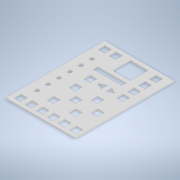
# Autodesk Inventor part: Front Plywood
Saved by Autodesk Inventor 2021.1 (Build 251245000, 245)
## iProperties
Created: 2020-08-02
Part Number: Front Plywood
Material: Generic
Document SubType Name: Modeling
Designer: adick
Density: 1 g/cm^3
Appearance: Default
Author: adick
Autodesk Inventor part; units mm, degrees
ref_plane "YZ Plane" through (0, 0, 0) normal (1, 0, 0) x (0, 1, 0)
ref_plane "XZ Plane" through (0, 0, 0) normal (0, 1, 0) x (-1, 0, 0)
ref_plane "XY Plane" through (0, 0, 0) normal (0, 0, 1) x (1, 0, 0)
sketch "Sketch1" plane through (0, 0, 0) normal (0, 1, 0) x (-1, 0, 0)
  line L0 (0, 0) -> (190, 0)
  line L1 (190, 0) -> (190, -270)
  line L2 (190, -270) -> (0, -270)
  line L3 (0, -270) -> (0, 0)
  line L4 (180, -10) -> (160, -10)
  line L5 (160, -10) -> (160, -30)
  line L6 (160, -30) -> (180, -30)
  line L7 (180, -30) -> (180, -10)
  line L8 (150, -10) -> (130, -10)
  line L9 (130, -10) -> (130, -30)
  line L10 (130, -30) -> (150, -30)
  line L11 (150, -30) -> (150, -10)
  line L12 (120, -10) -> (100, -10)
  line L13 (100, -10) -> (100, -30)
  line L14 (100, -30) -> (120, -30)
  line L15 (120, -30) -> (120, -10)
  line L16 (90, -10) -> (70, -10)
  line L17 (70, -10) -> (70, -30)
  line L18 (70, -30) -> (90, -30)
  line L19 (90, -30) -> (90, -10)
  line L20 (60, -10) -> (40, -10)
  line L21 (40, -10) -> (40, -30)
  line L22 (40, -30) -> (60, -30)
  line L23 (60, -30) -> (60, -10)
  line L24 (28.2524, -10) -> (8.2524, -10)
  line L25 (8.2524, -10) -> (8.2524, -30)
  line L26 (8.2524, -30) -> (28.2524, -30)
  line L27 (28.2524, -30) -> (28.2524, -10)
  circle A0 centre (165, -60) radius 6
  circle A1 centre (165, -90) radius 6
  circle A2 centre (165, -120) radius 6
  circle A3 centre (165, -150) radius 6
  circle A4 centre (165, -180) radius 6
  circle A5 centre (165, -210) radius 6
  line L28 (180, -260) -> (160, -260)
  line L29 (160, -260) -> (160, -240)
  line L30 (160, -240) -> (180, -240)
  line L31 (180, -240) -> (180, -260)
  line L32 (150, -260) -> (130, -260)
  line L33 (130, -260) -> (130, -240)
  line L34 (130, -240) -> (150, -240)
  line L35 (150, -240) -> (150, -260)
  line L36 (130, -50) -> (110, -50)
  line L37 (110, -50) -> (110, -70)
  line L38 (110, -70) -> (130, -70)
  line L39 (130, -70) -> (130, -50)
  line L40 (100, -80) -> (80, -80)
  line L41 (80, -80) -> (80, -100)
  line L42 (80, -100) -> (100, -100)
  line L43 (100, -100) -> (100, -80)
  line L44 (70, -70) -> (50, -70)
  line L45 (50, -70) -> (50, -50)
  line L46 (50, -50) -> (70, -50)
  line L47 (70, -50) -> (70, -70)
  line L48 (70, -110) -> (50, -110)
  line L49 (50, -110) -> (50, -130)
  line L50 (50, -130) -> (70, -130)
  line L51 (70, -130) -> (70, -110)
  line L52 (40, -80) -> (20, -80)
  line L53 (20, -80) -> (20, -100)
  line L54 (20, -100) -> (40, -100)
  line L55 (40, -100) -> (40, -80)
  line L56 (110, -110) -> (130, -110)
  line L57 (130, -110) -> (130, -130)
  line L58 (130, -130) -> (110, -130)
  line L59 (110, -130) -> (110, -110)
  line L60 (20, -260) -> (40, -260)
  line L61 (40, -260) -> (40, -240)
  line L62 (40, -240) -> (20, -240)
  line L63 (20, -240) -> (20, -260)
  line L64 (40, -230) -> (20, -230)
  line L65 (20, -230) -> (20, -210)
  line L66 (20, -210) -> (40, -210)
  line L67 (40, -210) -> (40, -230)
  line L68 (20, -200) -> (40, -200)
  line L69 (40, -200) -> (40, -180)
  line L70 (40, -180) -> (20, -180)
  line L71 (20, -180) -> (20, -200)
  line L72 (20, -170) -> (40, -170)
  line L73 (40, -170) -> (40, -150)
  line L74 (40, -150) -> (20, -150)
  line L75 (20, -150) -> (20, -170)
  line L76 (60, -260) -> (110, -260)
  line L77 (110, -260) -> (110, -210)
  line L78 (110, -210) -> (60, -210)
  line L79 (60, -210) -> (60, -260)
  line L80 (60, -200) -> (140, -200)
  line L81 (140, -200) -> (140, -186)
  line L82 (140, -186) -> (60, -186)
  line L83 (60, -186) -> (60, -200)
  line L84 (70, -170) -> (70, -150)
  line L85 (80, -150) -> (80, -170)
  line L86 (110, -170) -> (130, -170)
  line L87 (130, -170) -> (130, -150)
  line L88 (130, -150) -> (110, -150)
  line L89 (110, -150) -> (110, -170)
  line L90 (70, -150) -> (50, -160)
  line L91 (70, -170) -> (50, -160)
  line L92 (80, -150) -> (100, -160)
  line L93 (80, -170) -> (100, -160)
  constraints: 188 end point, 44 parallel, 22 horizontal, 22 perpendicular, 16 point on line, 6 centre point
extrude "Extrusion1" add sketch "Sketch1" along normal blind 3.175
body "Solid1"
